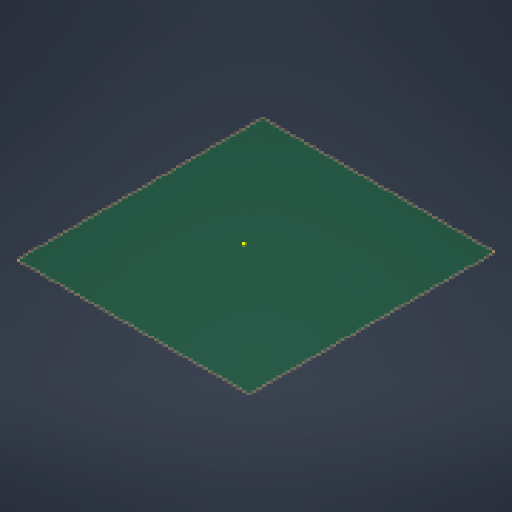
# Autodesk Inventor part: upper_middle_gasket
Saved by Autodesk Inventor 2026.2 (Build 302298000, 298)
## iProperties
Created: 2026-04-07
Part Number: upper_middle_gasket
Material: Generic
Document SubType Name: Modeling
Designer: Tathagata Sikdar
Density: 1 g/cm^3
Appearance: Default
Author: Tathagata Sikdar
Autodesk Inventor part; units mm, degrees
ref_plane "YZ Plane" through (0, 0, 0) normal (1, 0, 0) x (0, 1, 0)
ref_plane "XZ Plane" through (0, 0, 0) normal (0, 1, 0) x (-1, 0, 0)
ref_plane "XY Plane" through (0, 0, 0) normal (0, 0, 1) x (1, 0, 0)
ref_plane "Work Plane1" through (13.0846, 63.2868, -7.3851) normal (0, -1, 0) x (1, 0, 0)
sketch "Sketch1" plane through (13.0846, 63.2868, -7.3851) normal (0, -1, 0) x (1, 0, 0)
  circle A0 centre (0, -1.0676) radius 67.3144 construction
  circle A1 centre (0, -1.0676) radius 65.3144 construction
  arc A2 (21.565, -71.3061) -> (41.0886, -67.5378) centre (26.3661, -43.7208) ccw construction
  arc A3 (21.565, -71.3061) -> (-21.565, -71.3061) centre (0, -1.0676) ccw construction
  arc A4 (-41.0886, -67.5378) -> (-21.565, -71.3061) centre (-26.3661, -43.7208) ccw construction
  arc A5 (-78.1444, -1.0676) -> (-41.0886, -67.5378) centre (0, -1.0676) ccw construction
  line L0 (-78.1444, -1.0676) -> (-78.1444, 85.0131) construction
  line L1 (-78.1444, 85.0131) -> (-69.4624, 93.6951) construction
  line L2 (-69.4624, 93.6951) -> (69.4624, 93.6951) construction
  line L3 (69.4624, 93.6951) -> (78.1444, 85.0131) construction
  line L4 (78.1444, 85.0131) -> (78.1444, -1.0676) construction
  arc A6 (41.0886, -67.5378) -> (78.1444, -1.0676) centre (0, -1.0676) ccw construction
  arc A7 (14.16, -71.1254) -> (42.1402, -69.239) centre (26.3661, -43.7208) ccw construction
  arc A8 (42.1402, -69.239) -> (80.1444, -1.0676) centre (0, -1.0676) ccw construction
  line L5 (80.1444, -1.0676) -> (80.1444, 85.8416) construction
  line L6 (80.1444, 85.8416) -> (70.2909, 95.6951) construction
  line L7 (70.2909, 95.6951) -> (-70.2909, 95.6951) construction
  line L8 (-70.2909, 95.6951) -> (-80.1444, 85.8416) construction
  line L9 (-80.1444, 85.8416) -> (-80.1444, -1.0676) construction
  arc A9 (-80.1444, -1.0676) -> (-42.1402, -69.239) centre (0, -1.0676) ccw construction
  arc A10 (-42.1402, -69.239) -> (-14.16, -71.1254) centre (-26.3661, -43.7208) ccw construction
  arc A11 (14.16, -71.1254) -> (-14.16, -71.1254) centre (0, -1.0676) ccw construction
  circle A12 centre (0, -1.0676) radius 69.3944
  point P0 (-13.0846, 7.3851)
  point P1 (-69.3944, -1.0676)
  dimension "d0" = 2.08
  constraints: 2 horizontal alignment, 1 coincident, 2 other
ref_plane "Work Plane2" through (-56.3098, 63.2868, -8.4527) normal (0, 0, -1) x (-1, 0, 0)
sketch "Sketch2" plane through (-56.3098, 63.2868, -8.4527) normal (0, 0, -1) x (-1, 0, 0)
  circle A0 centre (0, 0) radius 2.5
  point P0 (-56.3098, -63.2868)
  dimension "d1" = 5
  constraints: 1 centre point, 1 coincident
  measures "d1" diameter of A0
sweep "Sweep1" add profiles "Sketch2" path "Sketch1"
body "Solid1"
